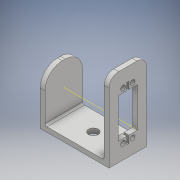
# Autodesk Inventor part: ShoulderPart1
Saved by Autodesk Inventor 2018 (Build 220112000, 112)
## iProperties
Created: 2018-02-08
Part Number: ShoulderPart1
Material: Générique
Document SubType Name: Modeling
Designer: Thomas
Density: 1 g/cm^3
Appearance: Par défaut
Author: Thomas
Autodesk Inventor part; units mm, degrees
ref_plane "YZ Plane" through (0, 0, 0) normal (1, 0, 0) x (0, 1, 0)
ref_plane "XZ Plane" through (0, 0, 0) normal (0, 1, 0) x (-1, 0, 0)
ref_plane "XY Plane" through (0, 0, 0) normal (0, 0, 1) x (1, 0, 0)
sketch "Esquisse1" plane through (0, 0, 0) normal (0, 0, 1) x (1, 0, 0)
  line L0 (0, 0) -> (-71.5, 0)
  line L1 (-71.5, 0) -> (-71.5, 39)
  line L2 (-71.5, 39) -> (0, 39)
  line L3 (0, 39) -> (0, 0)
  dimension "d0" = 71.5
  dimension "d1" = 39
  constraints: 8 end point, 2 parallel, 1 horizontal, 1 perpendicular
  measures "d0" distance of L0.start L0.end
  measures "d1" distance of L0.end L1.end
extrude "Extrusion1" add sketch "Esquisse1" along normal blind 5
sketch "Esquisse2" plane through (0, 0, 5) normal (0, 0, 1) x (1, 0, 0)
  line L0 (0, 39) -> (-71.5, 39) projected
  line L1 (-71.5, 39) -> (0, 0)
  line L2 (0, 0) -> (0, 39) projected
  line L3 (-71.5, 0) -> (0, 39)
  circle A0 centre (-35.75, 19.5) radius 5
  dimension "d4" = 10
  constraints: 4 end point, 2 midpoint, 1 centre point, 1 coincident
  measures "d4" diameter of A0
extrude "Extrusion2" cut sketch "Esquisse2" against normal blind 5 contours A0 L1 L3 | L3 L1 A0 | L1 L3 A0 | A0 L3 L1
sketch "Esquisse3" plane through (-71.5, 0, 0) normal (-1, 0, 0) x (0, 0, 1)
  line L0 (0, 39) -> (5, 39) projected
  line L1 (5, 39) -> (54.4, 39)
  line L2 (54.4, 39) -> (54.4, 0)
  line L3 (54.4, 0) -> (5, 0)
  line L4 (5, 0) -> (5, 39)
  point P0 (0, 0)
  dimension "d7" = 49.4
  constraints: 8 end point, 2 parallel, 1 horizontal, 1 perpendicular
  measures "d7" distance of L2.end L3.end
extrude "Extrusion3" add sketch "Esquisse3" against normal blind 5
fillet "Congé1" radius 18 1 edges at (-69, 0, 54.4)
fillet "Congé2" radius 18 1 edges at (-69, 39, 54.4)
sketch "Esquisse4" plane through (-71.5, 0, 0) normal (-1, 0, 0) x (0, 0, 1)
  line L0 (36.4, 0) -> (5, 0) projected
  line L1 (5, 0) -> (54.4, 39)
  line L2 (5, 39) -> (5, 0) projected
  line L3 (5, 39) -> (54.4, 0)
  circle A0 centre (29.7, 19.5) radius 5
  point P0 (0, 0)
  dimension "d12" = 10
  constraints: 4 end point, 1 centre point, 1 coincident, 1 midpoint
  measures "d12" diameter of A0
extrude "Extrusion4" add sketch "Esquisse4" along normal blind 10 contours A0 L3 L1 | L1 L3 A0 | L3 A0 L1 | L1 A0 L3
sketch "Esquisse5" plane through (0, 0, 0) normal (1, 0, 0) x (0, 0, -1)
  line L0 (-5, 0) -> (-81.9, 0)
  line L1 (-81.9, 0) -> (-81.9, 39)
  line L2 (-81.9, 39) -> (-5, 39)
  line L3 (-5, 39) -> (-5, 0)
  point P0 (0, 0)
  point P1 (-36.4, 39)
  dimension "d15" = 76.9
  dimension "d16" = 39
  constraints: 8 end point, 2 parallel, 1 horizontal, 1 perpendicular
  measures "d15" distance of L1.end L2.end
  measures "d16" distance of L2.end L0.start
extrude "Extrusion5" add sketch "Esquisse5" against normal blind 5
fillet "Congé3" radius 10 1 edges at (-2.5, 39, 81.9)
fillet "Congé4" radius 10 1 edges at (-2.5, 0, 81.9)
sketch "Esquisse6" plane through (0, 0, 0) normal (1, 0, 0) x (0, 0, -1)
  line L0 (-60.501, 9.5) -> (-19.501, 9.5)
  line L1 (-19.501, 29.5) -> (-60.501, 29.5)
  circle A0 centre (-15.111, 14.5) radius 2.5
  circle A1 centre (-15.111, 24.5) radius 2.5
  circle A2 centre (-64.891, 14.5) radius 2.5
  circle A3 centre (-64.891, 24.5) radius 2.5
  line L2 (-19.501, 18.5) -> (-12.001, 18.5)
  line L3 (-12.001, 18.5) -> (-12.001, 20.5)
  line L4 (-12.001, 20.5) -> (-19.501, 20.5)
  line L5 (-60.501, 18.5) -> (-68.001, 18.5)
  line L6 (-68.001, 18.5) -> (-68.001, 20.5)
  line L7 (-68.001, 20.5) -> (-60.501, 20.5)
  line L8 (-19.501, 9.5) -> (-19.501, 18.5)
  line L9 (-19.501, 20.5) -> (-19.501, 29.5)
  line L10 (-60.501, 9.5) -> (-60.501, 18.5)
  line L11 (-60.501, 20.5) -> (-60.501, 29.5)
  line L12 (0, 0) -> (-71.9, 0) projected
  line L13 (0, 39) -> (-71.9, 39) projected
  line L14 (0, 39) -> (0, 0) projected
  point P0 (-29.706, 19.5075)
  dimension "d21" = 41
  dimension "d22" = 20
  dimension "d23" = 5
  dimension "d24" = 5
  dimension "d25" = 5
  dimension "d26" = 5
  dimension "d27" = 10
  dimension "d29" = 5
  dimension "d30" = 10
  dimension "d31" = 5
  dimension "d33" = 9
  dimension "d34" = 9
  dimension "d35" = 9
  dimension "d36" = 9
  dimension "d37" = 7.5
  dimension "d38" = 7.5
  dimension "d40" = 9.5
  dimension "d41" = 9.5
  dimension "d42" = 4.39
  dimension "d43" = 4.39
  dimension "d44" = 10.205
  dimension "d49" = 29.706
  dimension "d50" = 41
  dimension "d51" = 4.39
  dimension "d52" = 4.39
  constraints: 24 end point, 6 equal length, 4 centre point, 3 horizontal, 2 perpendicular, 1 vertical
  measures "d21" distance of L1.start L1.end
  measures "d22" distance of L0.end L1.start
  measures "d23" diameter of A0
  measures "d24" diameter of A1
  measures "d25" diameter of A2
  measures "d26" diameter of A3
  measures "d27" distance of A1.centre A0.centre
  measures "d29" distance from line of L0 A0.centre
  measures "d30" distance of A3.centre A2.centre
  measures "d31" distance from line of L1 A3.centre
  measures "d33" distance of L0.start L5.start
  measures "d34" distance of L7.end L1.end
  measures "d35" distance of L0.end L2.start
  measures "d36" distance of L4.end L1.start
  measures "d37" distance of L3.end L4.end
  measures "d38" distance of L6.end L7.end
  measures "d40" distance between parallel lines of L0 L12
  measures "d41" distance between parallel lines of L13 L1
  measures "d42" distance from line of L8 A0.centre
  measures "d43" distance from line of L9 A1.centre
  measures "d44" distance from line of L8 point (-29.706, 19.508)
  measures "d49" distance from line of L14 point (-29.706, 19.508)
  measures "d50" distance of L0.start L0.end
  measures "d51" distance from line of L10 A2.centre
  measures "d52" distance from line of L11 A3.centre
extrude "Extrusion6" cut sketch "Esquisse6" against normal blind 5
fillet "Congé5" radius 2 1 edges at (-66.5, 19.5, 5)
fillet "Congé6" radius 2 1 edges at (-5, 19.5, 5)
